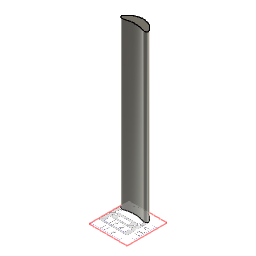
lens (Autodesk Fusion 360 design; units mm, degrees)
Autodesk Fusion 360 part; units mm, degrees
sketch "Esquisse1" plane through (0, 0, 0) normal (0, 0, 1) x (1, 0, 0)
  spline S0 degree 5 poles (-10.9, 6.9) (-10.885, 6.9401) (-10.8456, 7.0267) (-10.7585, 7.1783) (-10.5896, 7.4277) (-10.3068, 7.8068) (-9.9736, 8.2279) (-9.6124, 8.6592) (-9.2433, 9.0697) (-8.88, 9.4373) (-8.5268, 9.7546) (-8.1813, 10.0244) (-7.8366, 10.2565) (-7.4832, 10.4639) (-7.1116, 10.6589) (-6.7144, 10.8495) (-6.2876, 11.0371) (-5.8303, 11.2187) (-5.3443, 11.3884) (-4.8338, 11.5387) (-4.3046, 11.6626) (-3.7648, 11.7545) (-3.2232, 11.8126) (-2.6895, 11.8372) (-2.1726, 11.8309) (-1.6801, 11.7974) (-1.2174, 11.7409) (-0.7866, 11.6655) (-0.3856, 11.5744) (-0.0082, 11.4693) (0.3534, 11.3515) (0.707, 11.2213) (1.0586, 11.0787) (1.4102, 10.9237) (1.7591, 10.7562) (2.1003, 10.5762) (2.4279, 10.3842) (2.7374, 10.1808) (3.0273, 9.9674) (3.3003, 9.7455) (3.5611, 9.5171) (3.814, 9.2837) (4.0618, 9.0463) (4.3031, 8.8048) (4.5333, 8.5587) (4.7472, 8.3075) (4.9404, 8.0518) (5.1123, 7.7939) (5.267, 7.5382) (5.4072, 7.2893) (5.5299, 7.0504) (5.6201, 6.8212) (5.6488, 6.5971) (5.5881, 6.3747) (5.4245, 6.1556) (5.1727, 5.9517) (4.8652, 5.7801) (4.5384, 5.6578) (4.2221, 5.597) (3.9245, 5.5986) (3.6357, 5.6539) (3.3371, 5.7492) (3.0085, 5.8687) (2.6375, 5.9992) (2.2216, 6.131) (1.7644, 6.257) (1.2744, 6.3726) (0.7623, 6.475) (0.2393, 6.563) (-0.2854, 6.6362) (-0.8054, 6.6953) (-1.3162, 6.7408) (-1.8157, 6.7738) (-2.3035, 6.7948) (-2.7814, 6.8038) (-3.2525, 6.7999) (-3.7215, 6.781) (-4.1936, 6.7448) (-4.6733, 6.6887) (-5.1636, 6.6113) (-5.6647, 6.5122) (-6.1735, 6.3931) (-6.6821, 6.2582) (-7.1798, 6.114) (-7.655, 5.9689) (-8.0975, 5.8332) (-8.5001, 5.7185) (-8.8608, 5.6374) (-9.1849, 5.6037) (-9.4833, 5.6294) (-9.7663, 5.7197) (-10.0409, 5.8703) (-10.3046, 6.0608) (-10.5455, 6.2595) (-10.7464, 6.4387) (-10.8876, 6.5853) (-10.9385, 6.6922) (-10.9357, 6.7861) (-10.915, 6.8599) (-10.9, 6.9) knots 0 0 0 0 0 0 0.01052632 0.02105263 0.03157895 0.04210526 0.05263158 0.06315789 0.07368421 0.08421053 0.09473684 0.10526316 0.11578947 0.12631579 0.13684211 0.14736842 0.15789474 0.16842105 0.17894737 0.18947368 0.2 0.21052632 0.22105263 0.23157895 0.24210526 0.25263158 0.26315789 0.27368421 0.28421053 0.29473684 0.30526316 0.31578947 0.32631579 0.33684211 0.34736842 0.35789474 0.36842105 0.37894737 0.38947368 0.4 0.41052632 0.42105263 0.43157895 0.44210526 0.45263158 0.46315789 0.47368421 0.48421053 0.49473684 0.50526316 0.51578947 0.52631579 0.53684211 0.54736842 0.55789474 0.56842105 0.57894737 0.58947368 0.6 0.61052632 0.62105263 0.63157895 0.64210526 0.65263158 0.66315789 0.67368421 0.68421053 0.69473684 0.70526316 0.71578947 0.72631579 0.73684211 0.74736842 0.75789474 0.76842105 0.77894737 0.78947368 0.8 0.81052632 0.82105263 0.83157895 0.84210526 0.85263158 0.86315789 0.87368421 0.88421053 0.89473684 0.90526316 0.91578947 0.92631579 0.93684211 0.94736842 0.95789474 0.96842105 0.97894737 0.98947368 1 1 1 1 1 1
  point P0 (-9.3, 9)
  point P1 (-7.2328, 10.5927)
  point P2 (-4.302, 11.6546)
  point P3 (-1, 11.7)
  point P4 (0.9424, 11.1241)
  point P5 (2.6367, 10.2437)
  point P6 (3.9, 9.2)
  point P7 (4.9, 8.1)
  point P8 (5.5, 7.1)
  point P9 (5.5561, 6.3632)
  point P10 (4.4572, 5.6513)
  point P11 (3.2, 5.8)
  point P12 (0.6, 6.5)
  point P13 (-2.7, 6.8)
  point P14 (-5.7, 6.5)
  point P15 (-8.6, 5.7)
  point P16 (-9.9, 5.8)
  point P17 (-10.8, 6.5)
extrude "Extrusion1" add sketch "Esquisse1" along normal blind 100
